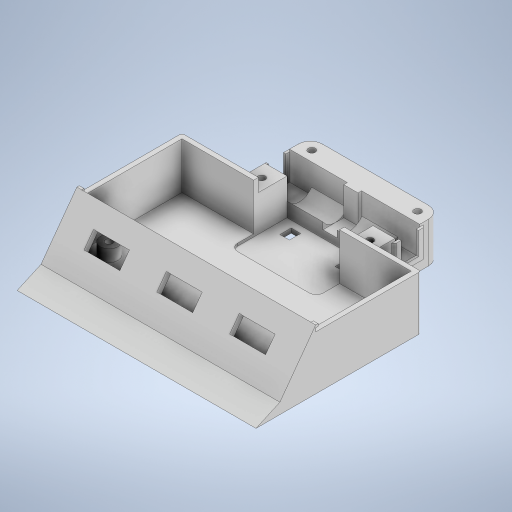
# Autodesk Inventor part: Sumec_telo_V4.1
Saved by Autodesk Inventor 2023.2 (Build 272271030, 271C)
## iProperties
Created: 2023-03-18
Part Number: Sumec_telo_V4.1
Material: Všeobecné
Document SubType Name: Modeling
Designer: jaryj
Density: 1 g/cm^3
Appearance: Výchozí
Author: jaryj
Autodesk Inventor part; units mm, degrees
ref_plane "YZ Plane" through (0, 0, 0) normal (1, 0, 0) x (0, 1, 0)
ref_plane "XZ Plane" through (0, 0, 0) normal (0, 1, 0) x (-1, 0, 0)
ref_plane "XY Plane" through (0, 0, 0) normal (0, 0, 1) x (1, 0, 0)
sketch "Náčrt1" plane through (0, 0, 0) normal (0, 1, 0) x (-1, 0, 0)
  line L0 (0, 0) -> (50, 0)
  line L1 (50, 0) -> (50, -69)
  line L2 (50, -69) -> (18, -69)
  line L3 (18, -69) -> (18, -81)
  line L4 (18, -81) -> (27.25, -81)
  line L5 (27.25, -81) -> (27.25, -69)
  line L6 (27.25, -81) -> (27.25, -91.25)
  line L7 (27.25, -91.25) -> (27.25, -100)
  line L8 (27.25, -100) -> (0, -100)
  line L9 (0, -100) -> (0, -91.25)
  line L10 (0, -91.25) -> (27.25, -91.25)
  line L11 (0, -91.25) -> (0, -81)
  line L12 (0, -81) -> (18, -81)
  line L13 (0, -81) -> (0, 0)
  line L14 (18, -69) -> (18, -57.25)
  line L15 (18, -57.25) -> (0, -57.25)
  line L16 (48, -25) -> (48, -67)
  line L17 (48, -67) -> (18, -67)
  line L18 (0, -25) -> (48, -25)
  dimension "d0" = 50
  dimension "d1" = 69
  dimension "d2" = 12
  dimension "d3" = 10.25
  dimension "d4" = 8.75
  dimension "d5" = 27.25
  dimension "d6" = 18
  dimension "d9" = 2
  dimension "d13" = 25
  dimension "d18" = 2
  dimension "d190" = 9.75
  constraints: 38 end point, 12 perpendicular, 7 point on line, 1 horizontal, 1 vertical
  measures "d0" distance of L0.start L0.end
  measures "d1" distance of L0.end L1.end
  measures "d2" distance of L4.end L5.end
  measures "d3" distance of L4.end L6.end
  measures "d4" distance of L6.end L7.end
  measures "d5" distance of L7.end L8.end
  measures "d6" distance of L3.end L11.end
  measures "d9" distance between parallel lines of L17 L2
  measures "d13" distance between parallel lines of L0 L18
  measures "d18" distance between parallel lines of L1 L16
  measures "d190" distance between parallel lines of L17 L15
extrude "Vysunutí1" add sketch "Náčrt1" along normal blind 3 contours L18 L16 L17 L14 L15 L13
extrude "Vysunutí2" add sketch "Náčrt1" along normal blind 1.888 contours L15 L14 L3 L12 L13
extrude "Vysunutí3" add sketch "Náčrt1" along normal blind 22.5 contours L0 L1 L2 L14 L17 L16 L18 L13
extrude "Vysunutí4" add sketch "Náčrt1" along normal blind 17 contours L5 L4 L3 L2 | L10 L7 L8 L9
extrude "Vysunutí15" add sketch "Náčrt1" along normal blind 5 contours L12 L4 L6 L10 L11
sketch "Náčrt2" plane through (-50, 0, -69) normal (-1, 0, 0) x (0, 0, 1)
  line L0 (69, 0) -> (69, 22.5) projected
  line L1 (69, 0) -> (59, 4.5)
  line L2 (0, 0) -> (69, 0) projected
  line L3 (44, 0) -> (44, 22.5)
  line L4 (44, 3) -> (44, 22.5) projected
  line L5 (44, 22.5) -> (44, 25)
  line L6 (44, 25) -> (59, 4.5)
  line L7 (0, 22.5) -> (69, 22.5) projected
  point P0 (45.8293, 22.5)
  dimension "d23" = 25
  dimension "d24" = 4.5
  dimension "d25" = 10
  constraints: 8 end point, 2 point on line, 1 vertical
  measures "d23" distance of L3.start L5.end
  measures "d24" distance from line of L2 L1.end
  measures "d25" horizontal distance of L0.start L1.end
extrude "Vysunutí5" cut sketch "Náčrt2" against normal through all contours L1 L6 L7 L0
extrude "Vysunutí6" add sketch "Náčrt2" against normal up to surface (50 mm away) contours L7 L5 L6
sketch "Náčrt3" plane through (0, 3, -25) normal (0, 0, -1) x (-1, 0, 0)
  line L0 (23, 15.167) -> (38, 15.167)
  line L1 (38, 15.167) -> (38, 0)
  line L2 (38, 0) -> (23, 0)
  line L3 (23, 0) -> (23, 15.167)
  line L4 (0, 15.167) -> (7.5, 15.167)
  line L5 (7.5, 15.167) -> (7.5, 0)
  line L6 (7.5, 0) -> (0, 0)
  line L7 (0, 0) -> (0, 15.167)
  line L8 (50, -3) -> (0, -3) projected
  dimension "d30" = 15
  dimension "d31" = 7.5
  dimension "d32" = 15.167
  dimension "d33" = 3
  dimension "d34" = 15.5
  constraints: 16 end point, 4 perpendicular, 4 point on line, 1 horizontal, 1 vertical alignment
  measures "d30" distance of L0.start L0.end
  measures "d31" distance of L4.start L4.end
  measures "d32" distance of L0.end L1.end
  measures "d33" distance between parallel lines of L8 L6
  measures "d34" distance between parallel lines of L3 L5
extrude "Vysunutí7" cut sketch "Náčrt3" against normal blind 9
sketch "Náčrt7" plane through (-48, 3, -67) normal (1, 0, 0) x (0, 0, -1)
  line L0 (-57, 1.5) -> (-42, 22) projected
  line L1 (-42, 15.167) -> (-42, 0) projected
  line L2 (-42, 0) -> (-50, 0)
  line L3 (-42, 0) -> (-51, 0) projected
  line L4 (-50, 0) -> (-50, 6.833)
  line L5 (-50, 6.833) -> (-42, 17.7664)
  line L6 (-42, 17.7664) -> (-42, 0)
  point P0 (-67, -3)
  point P1 (-38.3293, 19.5)
  point P2 (-36.5, 2)
  point P3 (-36.5, 2)
  dimension "d45" = 8
  dimension "d46" = 2.5
  constraints: 8 end point, 2 perpendicular, 1 collinear, 2 other
  measures "d45" distance of L2.start L2.end
extrude "Vysunutí9" cut sketch "Náčrt7" along normal through all
sketch "Náčrt11" plane through (-48, 22.5, -25) normal (0, 0, -1) x (-1, 0, 0)
  line L0 (2, -18) -> (2, 2.5) projected
  line L1 (2, 2.5) -> (0, 2.5)
  line L2 (0, 2.5) -> (0, 1.5)
  line L3 (0, 1.5) -> (2, 1.5)
  point P0 (-48, -22.5)
  point P1 (0, 0)
  point P2 (-2, 0)
  dimension "d69" = 1
  constraints: 6 end point, 2 perpendicular, 1 horizontal, 1 vertical alignment, 2 other
  measures "d69" distance of L1.end L2.end
extrude "Vysunutí13" add sketch "Náčrt11" along normal blind 1
sketch "Náčrt13" plane through (0, 17, 0) normal (0, 1, 0) x (1, 0, 0)
  line L0 (-18, 81) -> (-27.25, 81) projected
  line L1 (-27.25, 81) -> (-27.25, 69) projected
  point P0 (0, 0)
  point P1 (-22.625, 75)
  dimension "d84" = 6
  dimension "d85" = 4.625
  measures "d84" distance from line of L0 point (-22.625, 75)
  measures "d85" distance from line of L1 point (-22.625, 75)
hole "Díra2" at (-22.625, 17, -75) direction (0, -1, 0) diameter 3 depth 6
sketch "Náčrt14" plane through (0, 17, 0) normal (0, 1, 0) x (1, 0, 0)
  line L0 (-27.25, 100) -> (-27.25, 91.25) projected
  line L1 (0, 100) -> (-27.25, 100) projected
  point P0 (0, 0)
  point P1 (-22.125, 95.5)
  dimension "d93" = 5.125
  dimension "d101" = 4.5
  measures "d93" distance from line of L0 point (-22.125, 95.5)
  measures "d101" distance from line of L1 point (-22.125, 95.5)
hole "Díra3" at (-22.125, 17, -95.5) direction (0, -1, 0) diameter 3 depth 6
fillet "Zaoblení1" radius 3 1 edges at (-18, 2.444, -57.25)
fillet "Zaoblení2" radius 1 1 edges at (-50, 11.25, -69)
fillet "Zaoblení3" radius 5 1 edges at (-27.25, 8.5, -100)
sketch "Náčrt24" plane through (-18, 3, -67) normal (1, 0, 0) x (0, 0, -1)
  line L0 (24.25, 2) -> (24.25, 14) projected
  line L1 (24.25, 2) -> (14, 2) projected
  line L2 (14, 2) -> (14, 14) projected
  line L3 (14, 2) -> (24.25, 2) projected
  line L4 (24.25, 4.88) -> (24.25, 2)
  line L5 (24.25, 2) -> (14, 2)
  line L6 (14, 2) -> (14, 4.88)
  arc A0 (14, 4.88) -> (24.25, 4.88) centre (19.125, 8) ccw
  point P0 (-67, -3)
  point P1 (19.125, 2)
  dimension "d200" = 6
  constraints: 6 end point, 2 perpendicular, 2 point on circle, 2 point on line, 1 centre point, 1 horizontal alignment, 1 tangent
  measures "d200" radius of A0
extrude "Vysunutí22" add sketch "Náčrt24" along normal blind 15
sketch "Náčrt21" plane through (-27.25, 0, -69) normal (-1, 0, 0) x (0, 0, 1)
  line L0 (-20.75, 16) -> (-23.75, 16)
  line L1 (-22.25, 17) -> (-31, 17) projected
  line L2 (-23.75, 3.5) -> (-10.5, 3.5)
  line L3 (-10.5, 3.5) -> (-10.5, 16)
  line L4 (-10.5, 16) -> (-13.5, 16)
  line L5 (-13.5, 16) -> (-13.5, 6.5)
  line L6 (-13.5, 6.5) -> (-20.75, 6.5)
  line L7 (-20.75, 6.5) -> (-20.75, 16)
  line L8 (-23.75, 16) -> (-23.75, 3.5)
  line L9 (-22.25, 5) -> (-22.25, 17) projected
  line L10 (-22.25, 5) -> (-12, 5) projected
  line L11 (-12, 5) -> (-12, 17) projected
  line L12 (-12, 17) -> (0, 17) projected
  point P0 (69, 0)
  dimension "d172" = 1.5
  dimension "d173" = 1.5
  dimension "d174" = 1.5
  dimension "d175" = 1.5
  dimension "d176" = 1.5
  dimension "d177" = 1.5
  dimension "d180" = 1
  constraints: 12 end point, 3 perpendicular, 1 horizontal, 1 parallel, 1 vertical, 8 other
  measures "d172" distance between parallel lines of L7 L9
  measures "d173" distance between parallel lines of L6 L10
  measures "d174" distance between parallel lines of L5 L11
  measures "d175" distance between parallel lines of L11 L3
  measures "d176" distance between parallel lines of L2 L10
  measures "d177" distance between parallel lines of L8 L9
extrude "Vysunutí19" add sketch "Náčrt21" along normal blind 1
chamfer "Zkosení1" distance 1 angle 45 3 edges at (-28.25, 9.75, -92.75) (-28.25, 3.5, -86.125) (-28.25, 9.75, -79.5)
mirror "Zrcadlit1" about plane through (0, 0, -25) normal (1, 0, 0)
sketch "Náčrt16" plane through (0, 1.888, 0) normal (0, 1, 0) x (1, 0, 0)
  line L0 (-9.4, 73.375) -> (-13.4, 73.375)
  line L1 (-13.4, 73.375) -> (-13.4, 78.125)
  line L2 (-13.4, 78.125) -> (-9.4, 78.125)
  line L3 (-9.4, 78.125) -> (-9.4, 73.375)
  line L4 (-18, 69) -> (-18, 81) projected
  line L5 (13.75, 73.375) -> (9.75, 73.375)
  line L6 (9.75, 73.375) -> (9.75, 78.125)
  line L7 (9.75, 78.125) -> (13.75, 78.125)
  line L8 (13.75, 78.125) -> (13.75, 73.375)
  line L9 (18, 69) -> (18, 81) projected
  line L10 (-18, 81) -> (18, 81) projected
  point P0 (0, 0)
  dimension "d128" = 4
  dimension "d129" = 4.75
  dimension "d130" = 4.6
  dimension "d134" = 4.25
  dimension "d192" = 2.875
  constraints: 16 end point, 4 parallel, 2 equal length, 2 perpendicular, 1 horizontal, 1 horizontal alignment
  measures "d128" distance of L0.start L0.end
  measures "d129" distance of L2.end L0.start
  measures "d130" distance between parallel lines of L4 L1
  measures "d134" distance between parallel lines of L9 L8
  measures "d192" distance between parallel lines of L10 L2
extrude "Vysunutí16" cut sketch "Náčrt16" against normal through all
sketch "Náčrt17" plane through (0, 3, 0) normal (0, 1, 0) x (1, 0, 0)
  line L0 (-48, 17) -> (-38, 17) projected
  line L1 (-48, 17) -> (-48, 67) projected
  line L2 (48, 17) -> (38, 17) projected
  line L3 (48, 17) -> (48, 67) projected
  line L4 (-39.4, 19.625) -> (-43.4, 19.625)
  line L5 (-43.4, 19.625) -> (-43.4, 24.375)
  line L6 (-43.4, 24.375) -> (-39.4, 24.375)
  line L7 (-39.4, 24.375) -> (-39.4, 19.625)
  line L8 (42.75, 19.625) -> (38.75, 19.625)
  line L9 (38.75, 19.625) -> (38.75, 24.375)
  line L10 (38.75, 24.375) -> (42.75, 24.375)
  line L11 (42.75, 24.375) -> (42.75, 19.625)
  point P0 (0, 0)
  point P1 (-41.4, 19.625)
  point P2 (40.75, 19.625)
  dimension "d137" = 4
  dimension "d138" = 4.75
  dimension "d139" = 4.6
  dimension "d143" = 2.625
  dimension "d144" = 5.25
  dimension "d146" = 2.625
  constraints: 16 end point, 4 parallel, 2 equal length, 2 horizontal, 2 midpoint, 2 perpendicular
  measures "d137" distance of L4.start L4.end
  measures "d138" distance of L6.end L4.start
  measures "d139" distance between parallel lines of L1 L5
  measures "d143" distance between parallel lines of L0 L4
  measures "d144" distance between parallel lines of L3 L11
  measures "d146" distance from line of L2 point (40.75, 19.625)
extrude "Vysunutí17" cut sketch "Náčrt17" against normal through all
sketch "Náčrt18" plane through (0, 3, 0) normal (0, 1, 0) x (1, 0, 0)
  circle A0 centre (39.25, 59) radius 3.75
  circle A1 centre (-40.5, 29) radius 3.75
  line L0 (48, 67) -> (18, 67) projected
  line L1 (48, 25) -> (48, 67) projected
  line L2 (-48, 17) -> (-38, 17) projected
  line L3 (-48, 17) -> (-48, 67) projected
  point P0 (0, 0)
  point P1 (42.5, 67)
  dimension "d149" = 7.5
  dimension "d150" = 8
  dimension "d151" = 8.75
  dimension "d152" = 12
  dimension "d153" = 7.5
  constraints: 2 centre point, 1 equal radius
  measures "d149" diameter of A0
  measures "d150" distance from line of A0.centre L0
  measures "d151" distance from line of L1 A0.centre
  measures "d152" distance from line of L2 A1.centre
  measures "d153" distance from line of L3 A1.centre
extrude "Vysunutí18" add sketch "Náčrt18" along normal blind 5
sketch "Náčrt19" plane through (39.25, 8, -59) normal (0, 1, 0) x (1, 0, 0)
  circle A0 centre (0, 0) radius 3.75 projected
  point P0 (-39.25, -59)
  constraints: 1 coincident
hole "Díra4" at (39.25, 8, -59) direction (0, -1, 0) diameter 3 depth 6
sketch "Náčrt20" plane through (-40.5, 8, -29) normal (0, 1, 0) x (1, 0, 0)
  circle A0 centre (0, 0) radius 3.75 projected
  point P0 (40.5, -29)
  constraints: 1 coincident
hole "Díra5" at (-40.5, 8, -29) direction (0, -1, 0) diameter 3 depth 6
sketch "Náčrt25" plane through (-18, 7.88, -91.25) normal (0, 0, 1) x (1, 0, 0)
  line L0 (-4.25, 9.12) -> (40.25, 9.12) projected
  line L1 (15, 9.12) -> (21, 9.12)
  line L2 (21, 9.12) -> (21, -2.88)
  line L3 (21, -2.88) -> (15, -2.88)
  line L4 (15, -2.88) -> (15, 9.12)
  line L5 (15, 0) -> (15, -2.88) projected
  line L6 (21, 0) -> (21, -2.88) projected
  point P0 (18, -7.88)
  dimension "d203" = 12
  dimension "d204" = 6
  constraints: 8 end point, 2 parallel, 1 coincident, 1 horizontal, 1 perpendicular, 1 point on line
  measures "d203" distance of L3.end L1.start
  measures "d204" distance between parallel lines of L2 L4
extrude "Vysunutí23" add sketch "Náčrt25" along normal blind 1.5
